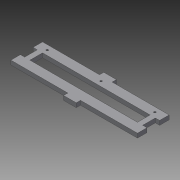
# Autodesk Inventor part: Controller_Back
Saved by Autodesk Inventor 2014 (Build 180170000, 170)
## iProperties
Created: 2014-11-10
Part Number: Controller_Back
Material: Generic
Document SubType Name: Modeling
Designer: ThatOtherGuy
Density: 1 g/cm^3
Appearance: Default
Author: ThatOtherGuy
Autodesk Inventor part; units mm, degrees
ref_plane "YZ Plane" through (0, 0, 0) normal (1, 0, 0) x (0, 1, 0)
ref_plane "XZ Plane" through (0, 0, 0) normal (0, 1, 0) x (-1, 0, 0)
ref_plane "XY Plane" through (0, 0, 0) normal (0, 0, 1) x (1, 0, 0)
sketch "Sketch1" plane through (0, 0, 0) normal (0, 0, 1) x (1, 0, 0)
  line L0 (0, 0) -> (200, 0)
  line L1 (200, 0) -> (200, 50)
  line L2 (200, 50) -> (0, 50)
  line L3 (0, 50) -> (0, 0)
  dimension "d0" = 200
  dimension "d1" = 50
  constraints: 8 end point, 2 parallel, 1 horizontal, 1 perpendicular
  measures "d0" distance of L0.start L0.end
  measures "d1" distance of L2.end L0.start
extrude "Extrusion1" add sketch "Sketch1" along normal blind 6.731
sketch "Sketch2" plane through (0, 0, 6.731) normal (0, 0, 1) x (1, 0, 0)
  line L0 (200, 50) -> (0, 50) projected
  line L1 (0, 50) -> (0, 0) projected
  line L2 (185, 15) -> (15, 15)
  line L3 (15, 15) -> (15, 35)
  line L4 (15, 35) -> (185, 35)
  line L5 (185, 35) -> (185, 15)
  circle A0 centre (15, 42.5) radius 1.588
  circle A1 centre (185, 42.5) radius 1.588
  circle A2 centre (100, 42.5) radius 1.588
  point P0 (100, 35)
  point P1 (100, 50)
  point P2 (15, 25)
  point P3 (0, 25)
  point P4 (0, 25)
  dimension "d4" = 20
  dimension "d6" = 15
  dimension "d15" = 3.176
  dimension "d18" = 50
  dimension "d23" = 7.5
  constraints: 8 end point, 5 midpoint, 4 vertical alignment, 3 centre point, 3 horizontal alignment, 2 equal radius, 2 parallel, 1 horizontal, 1 perpendicular
  measures "d4" distance of L2.end L3.end
  measures "d6" distance between parallel lines of L1 L3
  measures "d15" diameter of A2
  measures "d18" distance of L0.end L1.end
  measures "d23" distance from line of L0 A0.centre
extrude "Cutout" cut sketch "Sketch2" against normal up to next
sketch "Sketch3" plane through (0, 0, 6.731) normal (0, 0, 1) x (1, 0, 0)
  line L0 (200, 0) -> (200, 50) projected
  line L1 (0, 50) -> (0, 0) projected
  line L2 (0, 35) -> (6.731, 35)
  line L3 (6.731, 35) -> (6.731, 15)
  line L4 (6.731, 15) -> (0, 15)
  line L5 (0, 15) -> (0, 35)
  line L6 (200, 35) -> (193.269, 35)
  line L7 (193.269, 35) -> (193.269, 15)
  line L8 (193.269, 15) -> (200, 15)
  line L9 (200, 15) -> (200, 35)
  point P0 (193.269, 25)
  point P1 (200, 25)
  dimension "d9" = 20
  dimension "d10" = 6.731
  constraints: 16 end point, 4 parallel, 2 equal length, 2 horizontal, 2 midpoint, 2 perpendicular, 2 point on line, 1 collinear, 1 horizontal alignment
  measures "d9" distance of L6.end L7.end
  measures "d10" distance of L6.start L6.end
extrude "Tabs Neg" cut sketch "Sketch3" against normal up to next
sketch "Sketch4" plane through (0, 0, 6.731) normal (0, 0, 1) x (1, 0, 0)
  line L0 (6.731, 35) -> (6.731, 15) projected
  line L1 (6.731, 15) -> (0, 15) projected
  line L2 (0, 0) -> (200, 0) projected
  line L3 (90, 0) -> (110, 0)
  line L4 (110, 0) -> (110, -6.731)
  line L5 (110, -6.731) -> (90, -6.731)
  line L6 (90, -6.731) -> (90, 0)
  line L7 (200, 50) -> (0, 50) projected
  line L8 (90, 50) -> (110, 50)
  line L9 (110, 50) -> (110, 56.731)
  line L10 (110, 56.731) -> (90, 56.731)
  line L11 (90, 56.731) -> (90, 50)
  point P0 (100, -6.731)
  point P1 (100, 0)
  constraints: 16 end point, 4 equal length, 4 parallel, 2 horizontal, 2 midpoint, 2 perpendicular, 2 point on line, 1 collinear, 1 vertical alignment
extrude "Tabs Pos" add sketch "Sketch4" against normal blind 6.731
equation "\"d2\" = THICKB"
equation "\"d7\" = THICKB"
equation "\"d10\" = THICKB"
equation "\"d11\" = THICKB"
equation "\"d13\" = THICKB"
equation "\"THICKA\" = 3.175"
equation "\"THICKB\" = 6.731"
equation "\"THICKC\" = 12.7"
equation "\"THICKPLY\" = 5"
equation "\"MAGDIA\" = 9.5"
equation "\"BALLDIA\" = 12"
body "Solid1"
